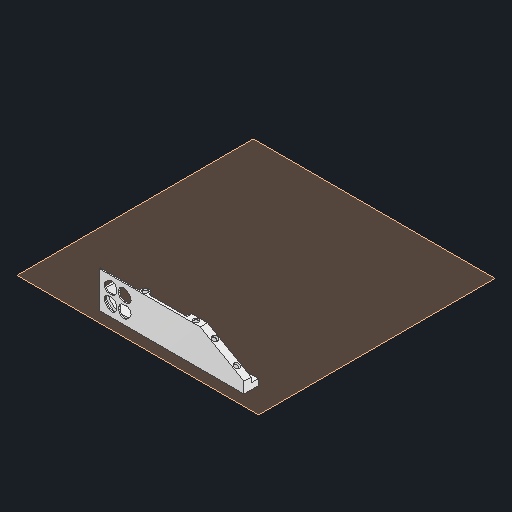
# Autodesk Inventor part: right_side
Saved by Autodesk Inventor 2023 (Build 270158000, 158)
## iProperties
Created: 2024-05-08
Part Number: right_side
Material: ABS Plastic
Document SubType Name: Modeling
Designer: szymo
Density: 1.06 g/cm^3
Appearance: Smooth - White
Mass: 11.6725 g
Surface Area: 103.74 cm^2
Volume: 11.0118 cm^3
Author: szymo
Autodesk Inventor part; units mm, degrees
ref_plane "YZ Plane" through (0, 0, 0) normal (1, 0, 0) x (0, 1, 0)
ref_plane "XZ Plane" through (0, 0, 0) normal (0, 1, 0) x (-1, 0, 0)
ref_plane "XY Plane" through (0, 0, 0) normal (0, 0, 1) x (1, 0, 0)
sketch "Sketch1" plane through (0, 0, 0) normal (0, 0, 1) x (1, 0, 0)
  line L0 (128, 8) -> (128, 3.5) projected
  line L1 (128, 3.5) -> (132, 3.5) projected
  line L2 (132, 3.5) -> (132, 0) projected
  line L3 (132, 0) -> (146, 0) projected
  line L4 (146, 0) -> (132, 9) projected
  line L5 (132, 9) -> (132, 8) projected
  line L6 (132, 8) -> (128, 8) projected
  circle A0 centre (-25, 12) radius 22.5 projected
  line L7 (116.5, 3.5) -> (116.5, 11.1395) projected
  line L8 (116.5, 14.6395) -> (116.5, 11.1395) projected
  line L9 (109.1155, 18.903) -> (116.5, 14.6395)
  line L10 (109.1155, 18.903) -> (83.8327, 33.5)
  line L11 (47.75, 33.5) -> (83.8327, 33.5) projected
  line L12 (0, 3.5) -> (0, 31) projected
  line L13 (0, 3.5) -> (0, 33.5)
  line L14 (0, 33.5) -> (83.8327, 33.5)
  line L15 (83.8327, 33.5) -> (128, 8)
  line L16 (128, 3.5) -> (0, 3.5)
  point P0 (0, 0)
  constraints: 12 end point, 2 collinear, 1 parallel, 1 point on line
extrude "Extrusion1" add sketch "Sketch1" against normal blind 2 contours L0 L16 L7 L8 L15 | L8 L7 L16 L12 L13 L14 L11 L10 L9
sketch "Sketch2" plane through (0, 0, -2) normal (0, 0, -1) x (-1, 0, 0)
  circle A0 centre (-15.375, 18.875) radius 13.7 projected
  line L0 (0, 33.5) -> (-83.8327, 33.5) projected
  line L1 (-128, 3.5) -> (0, 3.5) projected
  line L2 (-32.075, 33.5) -> (0, 33.5)
  line L3 (0, 33.5) -> (0, 3.5)
  line L4 (0, 3.5) -> (-32.075, 3.5)
  line L5 (-32.075, 3.5) -> (-32.075, 33.5)
  point P0 (0, 0)
  point P1 (-116.5, 3.5)
  dimension "d2" = 27.4
  dimension "d3" = 16.7
  constraints: 8 end point, 2 parallel, 1 horizontal, 1 perpendicular, 1 point on line
  measures "d2" diameter of A0
  measures "d3" distance from line of L5 A0.centre
extrude "Extrusion2" cut sketch "Sketch2" against normal blind 1 contours A0 | L3 L1 L5 L0
sketch "Sketch3" plane through (0, 0, -1) normal (0, 0, -1) x (-1, 0, 0)
  circle A0 centre (-15.375, 18.875) radius 13.7 projected
  line L0 (-32.075, 33.5) -> (0, 33.5) projected
  line L1 (-32.075, 3.5) -> (-32.075, 33.5) projected
  line L2 (0, 3.5) -> (-32.075, 3.5) projected
  line L3 (0, 33.5) -> (0, 3.5) projected
  line L4 (0, 3.5) -> (-128, 3.5) projected
  line L5 (0, 3.5) -> (-5, 3.5)
  line L6 (-5, 3.5) -> (-5, 6.5)
  line L7 (-5, 6.5) -> (0, 6.5)
  line L8 (0, 6.5) -> (0, 3.5)
  line L9 (-32.075, 3.5) -> (-27.075, 3.5)
  line L10 (-27.075, 3.5) -> (-27.075, 6.5)
  line L11 (-27.075, 6.5) -> (-32.075, 6.5)
  line L12 (-32.075, 6.5) -> (-32.075, 3.5)
  line L13 (-32.075, 9.5) -> (-25.365, 9.5)
  line L14 (-1.6801, 18.5) -> (0, 18.5)
  line L15 (0, 33.5) -> (0, 3.5) projected
  point P0 (0, 0)
  point P1 (-116.5, 3.5)
  point P2 (0, 18.5)
  dimension "d6" = 5
  dimension "d7" = 3
  dimension "d8" = 5
  dimension "d9" = 3
  dimension "d10" = 3
  constraints: 20 end point, 4 parallel, 3 perpendicular, 3 point on line, 2 horizontal, 2 point on circle, 1 midpoint
  measures "d6" distance of L6.end L7.end
  measures "d7" distance of L5.end L6.end
  measures "d8" distance of L11.end L10.end
  measures "d9" distance of L10.end L9.end
  measures "d10" distance between parallel lines of L13 L11
ref_plane "Work Plane1" through (1, 4.5, -18.6) normal (0, 0, 1) x (1, 0, 0)
ref_plane "Work Plane2" through (1.675, 5.175, -4.8) normal (0, 0, 1) x (1, 0, 0)
extrude "Extrusion3" add sketch "Sketch3" along normal blind 6.8 contours A0 L14 L3 L7 L6 L2 L10 L11 L1 L13 | L11 L10 L2 L1 | L3 L2 L6 L7
sketch "Sketch4" plane through (0, 0, -7.8) normal (0, 0, -1) x (-1, 0, 0)
  circle A0 centre (-15.375, 18.875) radius 13.7 projected
  line L0 (-1.6801, 18.5) -> (0, 18.5) projected
  line L1 (0, 33.5) -> (0, 18.5) projected
  line L2 (-32.075, 33.5) -> (0, 33.5) projected
  line L3 (-32.075, 9.5) -> (-32.075, 33.5) projected
  line L4 (-32.075, 9.5) -> (-25.365, 9.5) projected
  arc A1 (-25.365, 9.5) -> (-1.6801, 18.5) centre (-15.375, 18.875) ccw projected
  line L5 (-29.0741, 19.0336) -> (-32.075, 19.0336)
  line L6 (-32.075, 9.5) -> (-32.075, 33.5) projected
  line L7 (0, 18.5) -> (-1.6801, 18.5) projected
  line L8 (-1.6801, 18.5) -> (0, 18.5)
  arc A2 (-25.365, 9.5) -> (-1.6801, 18.5) centre (-15.375, 18.875) ccw projected
  line L9 (-25.365, 9.5) -> (-32.075, 9.5) projected
  line L10 (-32.075, 9.5) -> (-32.075, 3.5) projected
  line L11 (-32.075, 3.5) -> (0, 3.5) projected
  line L12 (0, 3.5) -> (0, 18.5) projected
  line L13 (0, 18.5) -> (-1.6801, 18.5) projected
  point P0 (0, 0)
  constraints: 4 end point, 1 collinear, 1 perpendicular, 1 point on line, 2 other
ref_plane "Work Plane3" through (1, 4.5, -18.6) normal (0, 0, 1) x (1, 0, 0)
extrude "Extrusion4" add sketch "Sketch4" along normal blind 5 contours A0 L4 L3 L5 | L0 L12 L11 L10 L4 A0
sketch "Sketch5" plane through (25.365, 9.5, -1) normal (0, 1, 0) x (1, 0, 0)
  line L0 (6.71, 0) -> (0, 0) projected
  line L1 (6.71, 1) -> (6.71, 0) projected
  line L2 (6.71, 1) -> (6.71, 6.8) projected
  line L3 (0, 6.8) -> (6.71, 6.8) projected
  line L4 (0, 0) -> (0, 6.8) projected
  line L5 (6.71, 0) -> (0, 6.8)
  line L6 (-0.1811, 0) -> (6.71, 6.8)
  point P0 (-25.365, -1)
  point P1 (3.2645, 3.4)
  constraints: 4 end point, 1 midpoint, 1 perpendicular, 1 point on line
hole "Hole1" at (28.6294, 9.5, -4.4) direction (0, -1, 0) diameter 3.6 end through all countersink diameter 6.5 countersink angle 90 clearance for "Countersunk Flat Head Screw ISO 2009/7046" size "M3" standard "ISO"
ref_plane "Work Plane4" through (41, 3.5, -89) normal (0, 1, 0) x (-1, 0, 0)
sketch "Sketch6" plane through (41, 3.5, -89) normal (0, 1, 0) x (-1, 0, 0)
  line L0 (8.925, 87) -> (-42.8327, 87) projected
  line L1 (-42.8327, 87) -> (-87, 87) projected
  line L2 (-87, 87) -> (8.925, 87) projected
  line L3 (-71, 89) -> (-71, 74) projected
  line L4 (-71, 74) -> (-87, 74) projected
  line L5 (-71, 87) -> (-64, 87)
  line L6 (-64, 87) -> (-64, 77)
  line L7 (-64, 77) -> (-71, 77)
  line L8 (-71, 77) -> (-71, 87)
  point P0 (41, 89)
  point P1 (-64, 87)
  dimension "d22" = 7
  dimension "d23" = 10
  constraints: 8 end point, 2 parallel, 2 point on line, 1 horizontal, 1 perpendicular
  measures "d22" distance of L6.end L7.end
  measures "d23" distance of L5.end L6.end
extrude "Extrusion5" add sketch "Sketch6" along normal blind 5
sketch "Sketch7" plane through (0, 0, -2) normal (0, 0, -1) x (-1, 0, 0)
  line L0 (-105, 8.5) -> (-105, 3.5) projected
  line L1 (-105, 3.5) -> (-32.075, 3.5) projected
  line L2 (-32.075, 3.5) -> (-32.075, 9.5) projected
  line L3 (-32.075, 9.5) -> (-32.075, 33.5) projected
  line L4 (-32.075, 33.5) -> (-83.8327, 33.5) projected
  line L5 (-83.8327, 33.5) -> (-128, 8) projected
  line L6 (-128, 8) -> (-128, 3.5) projected
  line L7 (-128, 3.5) -> (-112, 3.5) projected
  line L8 (-112, 3.5) -> (-112, 8.5) projected
  line L9 (-112, 8.5) -> (-105, 8.5) projected
  line L10 (-118.25, 3.5) -> (-115.75, 3.5) projected
  line L11 (-115.75, 3.5) -> (-118.25, 3.5)
  line L12 (-118.25, 3.5) -> (-118.25, 8.5)
  line L13 (-118.25, 8.5) -> (-115.75, 8.5)
  line L14 (-115.75, 8.5) -> (-115.75, 3.5)
  line L15 (-114, 3.5) -> (-120, 3.5)
  line L16 (-120, 3.5) -> (-120, 8.5)
  line L17 (-120, 8.5) -> (-114, 8.5)
  line L18 (-114, 8.5) -> (-114, 3.5)
  line L19 (-112, 8.5) -> (-114, 8.5)
  point P0 (0, 0)
  dimension "d26" = 5
  dimension "d27" = 6
  dimension "d28" = 1.75
  dimension "d29" = 1.75
  constraints: 18 end point, 4 parallel, 2 coincident, 2 horizontal, 2 perpendicular, 2 point on line, 1 collinear
  measures "d26" distance of L11.end L12.end
  measures "d27" distance of L16.end L17.end
  measures "d28" distance between parallel lines of L16 L12
  measures "d29" distance between parallel lines of L14 L18
extrude "Extrusion6" add sketch "Sketch7" along normal blind 10 contours L8 L7 L18 L19 | L18 L7 L14 L17 | L14 L7 L12 L13 | L12 L7 L16 L17
sketch "Sketch8" plane through (41, 8.5, -89) normal (0, 1, 0) x (1, 0, 0)
  line L0 (64, -77) -> (64, -87) projected
  line L1 (79, -87) -> (64, -87) projected
  line L2 (79, -87) -> (79, -77) projected
  line L3 (64, -77) -> (79, -77) projected
  line L4 (71, -77) -> (64, -83)
  line L5 (71, -89) -> (71, -74) projected
  point P0 (-41, -89)
  point P1 (67.5, -80)
  dimension "d40" = 4
  constraints: 3 point on line, 2 end point, 1 midpoint
  measures "d40" distance from line of L1 L4.end
hole "Hole2" at (108.5, 8.5, -9) direction (0, -1, 0) diameter 3.6 end through all countersink diameter 6 countersink angle 90 clearance for "Countersunk Flat Head Screw ISO 2009/7046" size "M3" standard "ISO"
sketch "Sketch9" plane through (0, 0, -2) normal (0, 0, -1) x (-1, 0, 0)
  line L0 (-120, 3.5) -> (-120, 8.5) projected
  line L1 (-120, 8.5) -> (-105, 8.5) projected
  line L2 (-105, 8.5) -> (-105, 3.5) projected
  line L3 (-105, 3.5) -> (-32.075, 3.5) projected
  line L4 (-32.075, 3.5) -> (-32.075, 9.5) projected
  line L5 (-32.075, 9.5) -> (-32.075, 33.5) projected
  line L6 (-32.075, 33.5) -> (-83.8327, 33.5) projected
  line L7 (-83.8327, 33.5) -> (-128, 8) projected
  line L8 (-128, 8) -> (-128, 3.5) projected
  line L9 (-128, 3.5) -> (-120, 3.5) projected
  line L10 (-70.8327, 33.5) -> (-122.7942, 3.5)
  line L11 (-105, 8.5) -> (-105, 13.7735)
  line L12 (0, 3.5) -> (-128, 3.5) projected
  line L13 (-128, 3.5) -> (-120, 3.5)
  line L14 (-120, 5.1132) -> (-120, 3.5)
  line L15 (-120, 5.1132) -> (-120, 8.5)
  line L16 (-120, 8.5) -> (-105, 8.5)
  line L17 (-122, 3.5) -> (-122, 11.4641)
  line L18 (-122, 3.5) -> (-114.0359, 3.5) construction
  line L19 (-32.075, 33.5) -> (0, 33.5) projected
  line L20 (-120, 8.5) -> (-120, 12.6188)
  line L21 (-70.8327, 33.5) -> (-32.075, 5.3538)
  line L22 (-72.2548, 32.6789) -> (-32.075, 3.5) construction
  line L23 (-73.6769, 31.8579) -> (-34.6277, 3.5)
  line L24 (-73.6769, 31.8579) -> (-73.6769, 3.5) construction
  line L25 (-75.1769, 30.9919) -> (-75.1769, 3.5)
  line L26 (-72.1769, 30.7686) -> (-72.1769, 3.5)
  line L27 (-75.1769, 3.5) -> (-96.0537, 18.9387) construction
  line L28 (-94.637, 19.7566) -> (-75.1769, 5.3656)
  line L29 (-97.4704, 18.1207) -> (-77.6997, 3.5)
  line L30 (-72.1769, 30.7686) -> (-51.9435, 3.5) construction
  line L31 (-72.1769, 28.2513) -> (-53.8113, 3.5)
  line L32 (-68.1265, 27.8271) -> (-50.0756, 3.5)
  line L33 (-105, 5.5) -> (-32.075, 5.5)
  line L34 (-32.075, 9.5) -> (-35.8782, 8.1157)
  line L35 (-39.2791, 6.8779) -> (-43.0649, 5.5)
  point P0 (0, 0)
  point P1 (-128, 5.75)
  point P2 (-77.6997, 3.5)
  point P3 (-72.1769, 3.5)
  point P4 (-34.6277, 3.5)
  point P5 (-50.0756, 3.5)
  point P6 (-53.8113, 3.5)
  point P7 (-37.3817, 5.5)
  point P8 (-51.5597, 5.5)
  point P9 (-55.2953, 5.5)
  point P10 (-72.1769, 5.5)
  point P11 (-80.4041, 5.5)
  point P12 (-32.2763, 5.5)
  dimension "d39" = 6.5
  dimension "d41" = 90
  dimension "d42" = 6
  dimension "d51" = 1.5
  dimension "d52" = 1.5
  dimension "d53" = 1.5
  dimension "d54" = 1.5
  dimension "d55" = 22.1042
  dimension "d56" = 25.3543
  dimension "d57" = 1.5
  dimension "d58" = 1.5
  dimension "d59" = 20.2335
  dimension "d60" = 17.3158
  dimension "d61" = 1.5
  dimension "d62" = 1.5
  dimension "d96" = 2
  dimension "d97" = 70
  constraints: 46 end point, 16 point on line, 6 parallel, 5 collinear, 5 perpendicular, 2 vertical, 1 horizontal, 1 midpoint, 21 other
  measures "d41" angle of L18 L17
  measures "d42" distance from line of L17 point (-128, 5.75)
  measures "d51" distance between parallel lines of L22 L21
  measures "d52" distance between parallel lines of L22 L23
  measures "d53" distance between parallel lines of L24 L26
  measures "d54" distance between parallel lines of L24 L25
  measures "d55" distance from line of L27 L25.start
  measures "d56" distance from line of L14.start L27
  measures "d57" distance between parallel lines of L27 L28
  measures "d58" distance between parallel lines of L27 L29
  measures "d59" distance of L26.end L30.end
  measures "d60" distance of L30.end L23.end
  measures "d61" distance between parallel lines of L30 L32
  measures "d62" distance between parallel lines of L30 L31
  measures "d97" angle of L34 L4
extrude "zeberka" add sketch "Sketch9" along normal blind 4 contours L2 L33 L29 L3 | L20 L7 L6 L10 L1 | L10 L11 L1 | L29 L33 L28 L25 L3 | L29 L10 L28 L33 | L25 L33 L26 L3 | L26 L33 L31 L3 | L21 L33 L23 L10 | L25 L10 L23 L26 L33 | L31 L33 L32 L3 | L34 L4 L33 L21 | L32 L33 L23 L3 | L31 L26 L23 L32 L33 | L21 L4 L3 L23 L33 | L33 L35 L23
sketch "Sketch11" plane through (0, 0, -2) normal (0, 0, -1) x (-1, 0, 0)
  line L0 (-32.075, 9.5) -> (-32.075, 33.5) projected
  line L1 (-32.075, 33.5) -> (-38.075, 33.5)
  line L2 (-38.075, 33.5) -> (-38.075, 27.5)
  line L3 (-38.075, 27.5) -> (-32.075, 27.5)
  line L4 (-32.075, 27.5) -> (-32.075, 33.5)
  point P0 (0, 0)
  dimension "d63" = 6
  dimension "d64" = 6
  constraints: 8 end point, 2 parallel, 1 horizontal, 1 perpendicular
  measures "d63" distance of L3.end L2.end
  measures "d64" distance of L2.end L1.end
extrude "Extrusion8" add sketch "Sketch11" along normal blind 4
fillet "Fillet1" radius 3 3 edges at (38.075, 30.5, -2) (38.075, 30.5, -6) (32.075, 30.5, -6)
chamfer "Chamfer1" distance 4 angle 45 2 edges at (39.575, 27.5, -2) (35.075, 27.5, -2)
sketch "Sketch13" plane through (0, 33.5, 0) normal (0, 1, 0) x (1, 0, 0)
  arc A0 (38.2466, 4) -> (35.4181, 6) centre (35.4181, 3) ccw projected
  line L0 (35.075, 6) -> (35.4181, 6) projected
  arc A1 (35.075, 6) -> (32.075, 3) centre (35.075, 3) ccw projected
  line L1 (32.075, 3) -> (32.075, 1) projected
  line L2 (32.075, 1) -> (0, 1) projected
  line L3 (0, 0) -> (0, 1) projected
  line L4 (83.8327, 0) -> (0, 0) projected
  line L5 (83.8327, 0) -> (83.8327, 6) projected
  line L6 (70.8327, 6) -> (83.8327, 6) projected
  line L7 (70.8327, 2) -> (70.8327, 6) projected
  line L8 (41.075, 2) -> (70.8327, 2) projected
  arc A2 (38.2466, 4) -> (41.075, 2) centre (41.075, 5) ccw projected
  line L9 (70.8327, 2) -> (70.8327, 0)
  line L10 (0, 0) -> (128, 0) projected
  constraints: 2 end point, 1 perpendicular, 1 point on line
extrude "Extrusion9" add sketch "Sketch13" against normal blind 5.75 contours L7 L6 L5 L4 L9
sketch "Sketch14" plane through (0, 33.5, 0) normal (0, 1, 0) x (1, 0, 0)
  line L0 (41.075, 2) -> (70.8327, 2) projected
  arc A0 (38.2466, 4) -> (41.075, 2) centre (41.075, 5) ccw projected
  arc A1 (38.2466, 4) -> (35.4181, 6) centre (35.4181, 3) ccw projected
  line L1 (35.075, 6) -> (35.4181, 6) projected
  arc A2 (35.075, 6) -> (32.075, 3) centre (35.075, 3) ccw projected
  line L2 (32.075, 3) -> (32.075, 1) projected
  line L3 (32.075, 1) -> (0, 1) projected
  line L4 (0, 0) -> (0, 1) projected
  line L5 (83.8327, 0) -> (0, 0) projected
  line L6 (83.8327, 0) -> (83.8327, 6) projected
  line L7 (70.8327, 6) -> (83.8327, 6) projected
  line L8 (70.8327, 2) -> (70.8327, 6) projected
  line L9 (70.8327, 6) -> (83.8327, 0)
  point P0 (0, 0)
  point P1 (35.2466, 3)
  point P2 (77.3327, 3)
  constraints: 2 end point, 1 midpoint
hole "Hole4" at (35.2466, 33.5, -3) at (77.3327, 33.5, -3) direction (0, -1, 0) diameter 4 depth 5 counterbore diameter 4.6 counterbore depth 1
sketch "Sketch15" plane through (128, 8, 0) normal (0.5, 0.8660254, 0) x (0.8660254, -0.5, 0)
  line L0 (0, 0) -> (-51, 0) projected
  line L1 (0, 0) -> (0, 2) projected
  line L2 (-9.2376, 2) -> (0, 2) projected
  line L3 (-9.2376, 2) -> (-9.2376, 6) projected
  line L4 (-51, 6) -> (-9.2376, 6) projected
  line L5 (-51, 0) -> (-51, 6) projected
  line L6 (-108.6013, 0) -> (2.25, 0) projected
  line L7 (-30.1188, 0) -> (-30.1188, 6)
  line L8 (-9.2376, 6) -> (-9.2376, 0)
  line L9 (-51, 6) -> (-30.1188, 0)
  line L10 (-30.1188, 6) -> (-51, 0)
  line L11 (-30.1188, 0) -> (-9.2376, 6)
  line L12 (-30.1188, 6) -> (-9.2376, 0)
  point P0 (-106.8513, 0)
  point P1 (-19.6782, 3)
  point P2 (-40.5594, 3)
  dimension "d87" = 20.8812
  dimension "d88" = 20.8812
  constraints: 12 end point, 3 midpoint, 2 parallel, 2 perpendicular, 2 point on line
  measures "d87" distance between parallel lines of L5 L7
  measures "d88" distance between parallel lines of L8 L7
hole "Hole5" at (110.9582, 17.8391, -3) at (92.8745, 28.2797, -3) direction (-0.5, -0.8660254, 0) diameter 4 depth 6 counterbore diameter 4.6 counterbore depth 2
sketch "Sketch16" plane through (0, 0, -2) normal (0, 0, -1) x (-1, 0, 0)
  line L0 (-120, 3.5) -> (-120, 12.6188) projected
  line L1 (-120, 12.6188) -> (-128, 8) projected
  line L2 (-128, 8) -> (-128, 3.5) projected
  line L3 (-128, 3.5) -> (-120, 3.5) projected
  point P0 (0, 0)
extrude "Extrusion10" cut sketch "Sketch16" against normal blind 2
sketch "Sketch18" plane through (0, 0, 0) normal (0, 0, 1) x (1, 0, 0)
  circle A0 centre (15.375, 18.875) radius 13.7 projected
  circle A1 centre (15.375, 18.875) radius 5 projected
  circle A2 centre (15.375, 18.875) radius 12.7
  line L0 (14.375, 32.575) -> (16.375, 32.575)
  line L1 (16.375, 32.575) -> (16.375, 5.175)
  line L2 (16.375, 5.175) -> (14.375, 5.175)
  line L3 (14.375, 5.175) -> (14.375, 32.575)
  line L4 (1.7115, 19.875) -> (29.075, 19.875)
  line L5 (29.075, 19.875) -> (29.075, 17.875)
  line L6 (29.075, 17.875) -> (1.7115, 17.875)
  line L7 (1.7115, 17.875) -> (1.7115, 19.875)
  arc A3 (10.476, 19.875) -> (14.375, 23.774) centre (10.3762, 23.8738) ccw
  arc A4 (16.375, 23.774) -> (20.274, 19.875) centre (20.3738, 23.8738) ccw
  arc A5 (20.274, 17.875) -> (16.375, 13.976) centre (20.3738, 13.8762) ccw
  arc A6 (14.375, 13.976) -> (10.476, 17.875) centre (10.3762, 13.8762) ccw
  point P0 (0, 0)
  point P1 (14.625, 14.3283)
  point P2 (10.7747, 17.875)
  point P3 (2.7144, 17.875)
  point P4 (14.375, 6.2144)
  point P5 (16.375, 6.2144)
  point P6 (28.0356, 17.875)
  point P7 (19.9753, 17.875)
  point P8 (16.125, 14.3283)
  point P9 (16.125, 23.4217)
  point P10 (19.9753, 19.875)
  point P11 (28.0356, 19.875)
  point P12 (16.375, 31.5356)
  point P13 (10.8283, 19.625)
  point P14 (14.375, 23.4753)
  point P15 (14.375, 31.5356)
  point P16 (2.7144, 19.875)
  point P17 (14.375, 19.875)
  point P18 (16.375, 19.875)
  point P19 (14.375, 17.875)
  point P20 (16.375, 17.875)
  point P21 (29.0385, 17.875)
  point P22 (29.075, 18.875)
  point P23 (29.0385, 19.875)
  point P24 (14.375, 5.2115)
  point P25 (15.375, 5.175)
  point P26 (16.375, 5.2115)
  dimension "d104" = 1
  dimension "d111" = 1
  dimension "d112" = 1
  dimension "d113" = 1
  dimension "d114" = 1
  dimension "d115" = 4
  dimension "d116" = 4
  dimension "d117" = 4
  dimension "d118" = 4
  constraints: 16 end point, 8 point on circle, 8 point on line, 5 centre point, 4 horizontal, 4 parallel, 2 perpendicular, 1 vertical, 11 other
  measures "d111" distance from line of A2.centre L1
  measures "d112" distance from line of L3 A2.centre
  measures "d113" distance from line of L4 A2.centre
  measures "d114" distance from line of point (15.375, 18.875) L6
  measures "d115" radius of A3
  measures "d116" radius of A4
  measures "d117" radius of A5
  measures "d118" radius of A6
extrude "Extrusion11" cut sketch "Sketch18" against normal up to next contours A2 L3 A1 L4 | L6 A1 L3 A2 | A3 L3 L4 | A1 A3 | A6 A1 | L6 L3 A6 | A2 L4 A1 L1 | L1 A1 L6 A2 | A4 L4 L1 | A1 A4 | A5 A1 | L1 L6 A5
fillet "Fillet2" radius 4 12 edges at (2.7144, 19.875, -0.5) (2.7144, 17.875, -0.5) (14.375, 6.2144, -0.5) (16.375, 6.2144, -0.5) (28.0356, 17.875, -0.5) (28.0356, 19.875, -0.5) (16.375, 31.5356, -0.5) (14.375, 31.5356, -0.5) (16.375, 19.875, -0.5) (16.375, 17.875, -0.5) (14.375, 17.875, -0.5) (14.375, 19.875, -0.5)
sketch "Sketch19" plane through (0, 3.5, -12.8) normal (0, -1, 0) x (1, 0, 0)
  line L0 (1.675, 8) -> (29.075, 8) projected
  line L1 (1.675, 8) -> (25.365, 8)
  line L2 (25.365, 8) -> (25.365, 10)
  line L3 (25.365, 10) -> (1.675, 10)
  line L4 (1.675, 10) -> (1.675, 8)
  line L5 (25.365, 11.8) -> (25.365, 5) projected
  point P0 (0, 12.8)
  dimension "d122" = 2
  constraints: 8 end point, 2 parallel, 1 collinear, 1 horizontal, 1 perpendicular
  measures "d122" distance of L2.end L1.end
extrude "Extrusion12" cut sketch "Sketch19" against normal blind 10
sketch "Sketch20" plane through (0, 3.5, -12.8) normal (0, -1, 0) x (1, 0, 0)
  circle A0 centre (117, 3.8) radius 1.25 projected
  point P0 (0, 12.8)
  constraints: 1 coincident
hole "Hole6" at (117, 3.5, -9) direction (0, 1, 0) diameter 3 depth 4 counterbore diameter 3.5 counterbore depth 1
equation "\"d28\" = d29"
equation "\"d52\" = d51"
equation "\"d54\" = d53"
equation "\"d58\" = d57"
equation "\"d62\" = d61"
equation "\"d87\" = d88"
body "Solid1"
